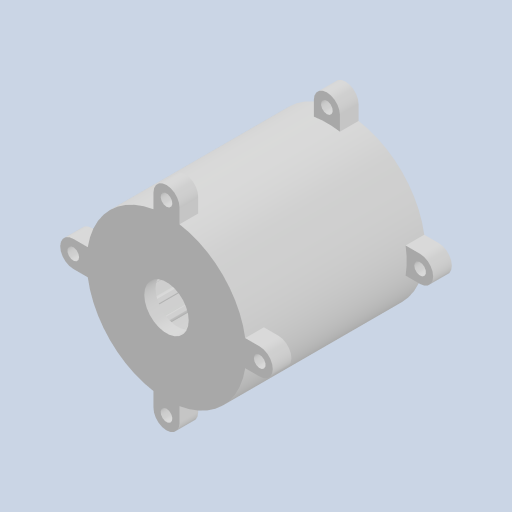
# Autodesk Inventor part: Inel_V2
Saved by Autodesk Inventor 2024 (Build 280153000, 153)
## iProperties
Created: 2023-12-13
Part Number: Inel_V2
Material: Generic
Document SubType Name: Modeling
Designer: mirun
Density: 1 g/cm^3
Appearance: Default
Author: mirun
Autodesk Inventor part; units mm, degrees
ref_plane "YZ Plane" through (0, 0, 0) normal (1, 0, 0) x (0, 1, 0)
ref_plane "XZ Plane" through (0, 0, 0) normal (0, 1, 0) x (-1, 0, 0)
ref_plane "XY Plane" through (0, 0, 0) normal (0, 0, 1) x (1, 0, 0)
sketch "Sketch1" plane through (0, 0, 0) normal (0, 0, 1) x (1, 0, 0)
  circle A0 centre (0, 0) radius 17.5 construction
  circle A1 centre (0, 0) radius 18.4
  circle A2 centre (0, 0) radius 16.8
  line L0 (0, 0) -> (0, 16.8)
  line L1 (0, 18.4) -> (0, 21.4)
  line L2 (0, 17.5) -> (0, 18.2)
  line L3 (0, 16.8) -> (0, 17.5)
  circle A3 centre (0, 0) radius 18.2 construction
  line L4 (0, 18.2) -> (0, 18.4)
  line L5 (-0.8, 18.3826) -> (-0.7913, 18.1828)
  arc A4 (-0.7913, 18.1828) -> (-0.45, 16.794) centre (1.7057, 18.0601) ccw
  line L6 (0.8, 18.3826) -> (0.7913, 18.1828)
  arc A5 (0.45, 16.794) -> (0.7913, 18.1828) centre (-1.7057, 18.0601) ccw
  circle A6 centre (0, 0) radius 21.4
  line L7 (0, 21.4) -> (0, 24.1252)
  point P0 (0.45, 16.794)
  dimension "d0" = 35
  dimension "d1" = 0.7
  dimension "d2" = 0.7
  dimension "d3" = 0.2
  dimension "d4" = 0.8
  dimension "d5" = 2.5
  dimension "d6" = 0.45
  dimension "d7" = 3
  constraints: 16 end point, 10 point on circle, 6 vertical, 5 centre point, 5 coincident, 4 symmetric about line, 2 vertical alignment, 1 line through centre, 5 other
  measures "d1" distance of L0.end L2.start
  measures "d2" distance of L2.start L2.end
  measures "d3" distance of L1.start L2.end
  measures "d4" horizontal distance of L1.start L5.start
  measures "d5" radius of A4
  measures "d6" horizontal distance of L0.end A2.end
  measures "d7" distance of L1.end L1.start
extrude "Extrusion1" add sketch "Sketch1" along normal blind 45 contours A6 | L6 A5 A2 L3 L2 L4 A1 | A1 L4 L2 L3 A2 A4 L5
pattern_circular "Circular Pattern1" count 28 over 360 about axis through (0, 0, 0) along (0, 0, 1) of "Extrusion1"
sketch "Sketch2" plane through (0, 0, 45) normal (0, 0, 1) x (1, 0, 0)
  circle A0 centre (0, 0) radius 21.4 construction
  arc A1 (-0.8, 18.3826) -> (-3.3106, 18.0997) centre (0, 0) ccw construction
  circle A2 centre (0, 0) radius 21.4
  circle A3 centre (0, 0) radius 5.95
  dimension "d15" = 11.9
  constraints: 2 centre point, 2 coincident, 1 concentric
  measures "d15" diameter of A3
extrude "Extrusion2" add sketch "Sketch2" along normal blind 3
sketch "Sketch3" plane through (0, 0, 48) normal (0, 0, 1) x (1, 0, 0)
  circle A0 centre (0, 0) radius 21.4 construction
  circle A1 centre (0, 0) radius 5.95 construction
  circle A2 centre (-25, 0.0008) radius 1.5625
  circle A3 centre (-25, 0.0008) radius 3.5
  line L0 (-25, -3.4992) -> (-21.112, -3.4992)
  line L1 (0, 0) -> (0, -32.0691)
  line L2 (0, 0) -> (-35.755, 0)
  line L3 (-25, 3.4992) -> (-21.112, 3.4992)
  circle A4 centre (0, 0) radius 21.4
  point P0 (-24.896, 3.4992)
  dimension "d17" = 7
  dimension "d16" = 3.125
  dimension "d18" = 25
  constraints: 8 end point, 3 horizontal, 2 centre point, 2 coincident, 2 symmetric about line, 1 perpendicular, 1 vertical, 5 other
  measures "d16" diameter of A2
  measures "d18" distance of point (0, 0) A2.centre
extrude "Extrusion3" add sketch "Sketch3" against normal blind 5 contours L2 A3 A2 | A2 L2 A3 | L2 A4 L0 A3 | A3 L3 A4 L2
pattern_circular "Circular Pattern2" count 4 over 360 about axis through (0, 0, 45) along (0, 0, 1) of "Extrusion3"
sketch "Sketch4" plane through (0, 0, 0) normal (0, 0, -1) x (-1, 0, 0)
  arc A0 (-0.8, 18.3826) -> (-3.3106, 18.0997) centre (0, 0) ccw construction
  circle A1 centre (0, 0) radius 21.4
  circle A2 centre (0, 0) radius 5.95 construction
  circle A3 centre (-25, 0) radius 1.5625
  circle A4 centre (-25, 0) radius 3.5
  line L0 (-25, -3.5) -> (-21.1118, -3.5)
  line L1 (0, 0) -> (0, -31.5162)
  line L2 (0, 0) -> (-42.9224, 0)
  line L3 (-25, 3.5) -> (-21.1118, 3.5)
  point P0 (-28.2794, -2.9463)
  point P1 (-28.2794, 4.0521)
  point P2 (-32.0634, 4.0521)
  dimension "d25" = 7
  dimension "d27" = 42.8
  dimension "d24" = 3.125
  dimension "d26" = 25
  constraints: 8 end point, 5 coincident, 3 horizontal, 2 centre point, 2 symmetric about line, 1 perpendicular, 1 point on line, 1 vertical, 8 other
  measures "d24" diameter of A3
  measures "d26" distance of point (0, 0) A3.centre
extrude "Extrusion4" add sketch "Sketch4" against normal blind 5 contours A1 L2 A4 L3 | A1 L0 A4 L2 | A4 L2 A3 | A4 L2 A3
pattern_circular "Circular Pattern3" count 4 over 360 about axis through (0, 0, 0) along (0, 0, 1) of "Extrusion4"
body "Solid1"
